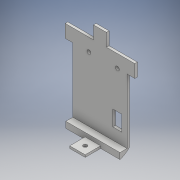
# Autodesk Inventor part: arm_1_case
Saved by Autodesk Inventor 2018 (Build 220112000, 112)
## iProperties
Created: 2018-02-06
Part Number: arm_1_case
Material: Genérico
Document SubType Name: Modeling
Designer: se_ma
Density: 1 g/cm^3
Appearance: Valor por defecto
Author: se_ma
Autodesk Inventor part; units mm, degrees
ref_plane "YZ Plane" through (0, 0, 0) normal (1, 0, 0) x (0, 1, 0)
ref_plane "XZ Plane" through (0, 0, 0) normal (0, 1, 0) x (-1, 0, 0)
ref_plane "XY Plane" through (0, 0, 0) normal (0, 0, 1) x (1, 0, 0)
sketch "Boceto1" plane through (0, 0, 0) normal (0, 1, 0) x (-1, 0, 0)
  line L0 (0, 0) -> (54, 0)
  line L1 (27, 10) -> (32, 10)
  line L2 (32, 10) -> (32, 0)
  line L3 (27, 10) -> (22, 10)
  line L4 (22, 10) -> (22, 0)
  line L5 (54, 0) -> (54, -10)
  line L6 (54, -10) -> (48, -10)
  line L7 (0, 0) -> (0, -10)
  line L8 (0, -10) -> (6, -10)
  line L9 (48, -10) -> (48, -60)
  line L10 (48, -60) -> (6, -60)
  line L11 (6, -60) -> (6, -10)
  dimension "d0" = 54
  dimension "d2" = 5
  dimension "d3" = 5
  dimension "d4" = 10
  dimension "d5" = 6
  dimension "d6" = 10
  dimension "d7" = 6
  dimension "d9" = 50
  constraints: 24 end point, 6 perpendicular, 3 vertical, 2 horizontal, 2 point on line
  measures "d0" distance of L0.start L0.end
  measures "d2" distance of L1.start L1.end
  measures "d3" distance of L1.start L3.end
  measures "d4" distance of L0.end L5.end
  measures "d5" distance of L5.end L6.end
  measures "d6" distance of L0.start L7.end
  measures "d7" distance of L7.end L8.end
  measures "d9" distance of L6.end L9.end
extrude "Extrusión1" add sketch "Boceto1" along normal blind 2 contours L0 L5 L6 L9 L10 L11 L8 L7
sketch "Boceto2" plane through (-48, 0, -60) normal (-1, 0, 0) x (0, 0, 1)
  line L0 (50, 2) -> (0, 2) projected
  line L1 (0, 2) -> (50, 2) projected
  line L2 (0, 0) -> (50, 0) projected
  line L3 (0, 2) -> (0, 0)
  arc A0 (0, 2) -> (0, -23) centre (11.5217, -10.5) ccw
  line L4 (0, 2) -> (0, -5.5)
  line L5 (0, -5.5) -> (-4.7264, -5.5)
  point P0 (60, 0)
  dimension "d15" = 25
  dimension "d16" = 17
  dimension "d27" = 7.5
  constraints: 6 end point, 3 perpendicular, 3 point on circle, 1 centre point
  measures "d15" distance of L0.end A0.end
  measures "d16" radius of A0
  measures "d27" distance of L0.end L4.end
sketch "Boceto3" plane through (0, 2, 0) normal (0, 1, 0) x (1, 0, 0)
  line L0 (-6, 10) -> (-13.5, 10)
  line L1 (-48, 10) -> (-35.576, 10)
  circle A0 centre (-35.576, 10) radius 1.5
  circle A1 centre (-13.5, 10) radius 1.5
  point P0 (0, 0)
  dimension "d19" = 7.5
  dimension "d20" = 12.424
  dimension "d21" = 3
  dimension "d22" = 3
  constraints: 4 end point, 2 centre point, 2 coincident, 2 horizontal
  measures "d19" distance of L0.start L0.end
  measures "d20" distance of L1.start L1.end
  measures "d21" diameter of A0
  measures "d22" diameter of A1
extrude "Extrusión3" cut sketch "Boceto3" against normal blind 2
extrude "Extrusión4" add sketch "Boceto2" against normal blind 42
sketch "Boceto5" plane through (-48, -5.5, -64.7264) normal (0, -1, 0) x (1, 0, 0)
  line L0 (0, 4.7264) -> (0, 54.7264) projected
  line L1 (0, 4.7264) -> (15, 4.7264)
  line L2 (42, 4.7264) -> (0, 4.7264) projected
  line L3 (42, 4.7264) -> (27, 4.7264)
  line L4 (15, 4.7264) -> (15, 1.7484)
  line L5 (15, 1.7484) -> (27, 1.7484)
  line L6 (27, 1.7484) -> (27, 4.7264)
  line L7 (15, 1.7484) -> (15, 0)
  line L8 (0, 0) -> (42, 0) projected
  line L9 (15, 0) -> (27, 0)
  line L10 (27, 0) -> (27, 1.7484)
  point P0 (48, 64.7264)
  dimension "d30" = 15
  dimension "d31" = 15
  dimension "d32" = 2.978
  constraints: 16 end point, 3 perpendicular, 3 point on line, 2 vertical, 1 horizontal
  measures "d30" distance of L0.start L1.end
  measures "d31" distance of L2.start L3.end
  measures "d32" distance of L1.end L4.end
extrude "Extrusión5" add sketch "Boceto5" along normal blind 12 contours L10 L8 L7 L5
sketch "Boceto6" plane through (-21, -5.5, -64.7264) normal (0, 0, -1) x (-1, 0, 0)
  line L0 (0, -12) -> (12, -12) projected
  line L1 (6, -12) -> (6, -6)
  circle A0 centre (6, -6) radius 1.5
  point P0 (-21, 5.5)
  dimension "d35" = 6
  dimension "d36" = 3
  constraints: 2 end point, 1 centre point, 1 coincident, 1 midpoint, 1 vertical
  measures "d35" distance of L1.start L1.end
  measures "d36" diameter of A0
extrude "Extrusión6" cut sketch "Boceto6" against normal blind 3
sketch "Boceto7" plane through (0, 2, 0) normal (0, 1, 0) x (1, 0, 0)
  line L0 (-54, 0) -> (0, 0) projected
  line L1 (-27, -10) -> (-32, -10)
  line L2 (-32, -10) -> (-32, 0)
  line L3 (-27, -10) -> (-22, -10)
  line L4 (-22, -10) -> (-22, 0)
  line L5 (-22, 0) -> (-32, 0)
  dimension "d40" = 5
  dimension "d41" = 5
  constraints: 10 end point, 3 point on line, 2 perpendicular, 1 collinear
  measures "d40" distance of L1.start L1.end
  measures "d41" distance of L1.start L3.end
extrude "Extrusión7" add sketch "Boceto7" against normal blind 2
sketch "Boceto8" plane through (0, 2, 0) normal (0, 1, 0) x (1, 0, 0)
  line L0 (-6, 60) -> (-6, 64.7264) projected
  line L1 (-6, 60) -> (-10, 60)
  line L2 (-6, 60) -> (-48, 60) projected
  line L3 (-10, 60) -> (-10, 51)
  line L4 (-10, 51) -> (-17, 51)
  line L5 (-17, 51) -> (-17, 39)
  line L6 (-17, 39) -> (-10, 39)
  line L7 (-10, 39) -> (-10, 51)
  point P0 (0, 0)
  dimension "d44" = 4
  dimension "d45" = 9
  dimension "d46" = 7
  dimension "d47" = 12
  constraints: 12 end point, 3 perpendicular, 1 collinear, 1 point on line, 1 vertical
  measures "d44" distance of L0.start L1.end
  measures "d45" distance of L1.end L3.end
  measures "d46" distance of L3.end L4.end
  measures "d47" distance of L4.end L5.end
extrude "Extrusión8" cut sketch "Boceto8" against normal blind 2
